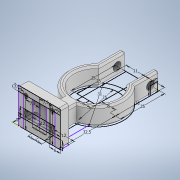
# Autodesk Inventor part: Endswitch Ender3 clamp
Saved by Autodesk Inventor 2020 (Build 240168000, 168)
## iProperties
Created: 2020-06-03
Part Number: Endswitch Ender3 clamp
Material: Generisch
Document SubType Name: Modeling
Designer: Daniel
Density: 1 g/cm^3
Appearance: Vorgabe
Author: Daniel
Autodesk Inventor part; units mm, degrees
ref_plane "YZ Plane" through (0, 0, 0) normal (1, 0, 0) x (0, 1, 0)
ref_plane "XZ Plane" through (0, 0, 0) normal (0, 1, 0) x (-1, 0, 0)
ref_plane "XY Plane" through (0, 0, 0) normal (0, 0, 1) x (1, 0, 0)
sketch "Skizze1" plane through (0, 0, 0) normal (0, 1, 0) x (-1, 0, 0)
  circle A0 centre (0, 0) radius 12.5
  line L0 (0, 0) -> (8, 0)
  line L1 (8, 0) -> (8, -25)
  line L2 (8, -25) -> (0, -25)
  line L3 (0, -25) -> (0, 0)
  line L4 (0, 0) -> (-8, 0)
  line L5 (-8, 0) -> (-8, -25)
  line L6 (-8, -25) -> (0, -25)
  line L7 (0, -25) -> (0, 0)
  line L8 (8, 0) -> (-8, 0)
  line L9 (-8, 0) -> (-8, 32.5)
  line L10 (-8, 32.5) -> (8, 32.5)
  line L11 (8, 32.5) -> (8, 0)
  line L12 (0, 32.5) -> (0, 27.5)
  line L13 (0, 27.5) -> (-12, 27.5)
  line L14 (-12, 27.5) -> (-12, 32.5)
  line L15 (-12, 32.5) -> (0, 32.5)
  line L16 (0, 32.5) -> (12, 32.5)
  line L17 (12, 32.5) -> (12, 27.5)
  line L18 (12, 27.5) -> (0, 27.5)
  line L19 (0, 27.5) -> (0, 32.5)
  circle A1 centre (0, 0) radius 15.5
  line L20 (0, 0) -> (11, 0)
  line L21 (11, 0) -> (11, -25)
  line L22 (11, -25) -> (0, -25)
  line L23 (0, -25) -> (0, 0)
  line L24 (0, 0) -> (-11, 0)
  line L25 (-11, 0) -> (-11, -25)
  line L26 (-11, -25) -> (0, -25)
  line L27 (0, -25) -> (0, 0)
  line L28 (0, 0) -> (4, 0)
  line L29 (4, 0) -> (4, 32.5)
  line L30 (4, 32.5) -> (0, 32.5)
  line L31 (0, 32.5) -> (0, 0)
  line L32 (0, 0) -> (-4, 0)
  line L33 (-4, 0) -> (-4, 32.5)
  line L34 (-4, 32.5) -> (0, 32.5)
  line L35 (0, 32.5) -> (0, 0)
  point P0 (8, -9.6047)
  point P1 (11, -10.9202)
  point P2 (4, 14.975)
  point P3 (4, 27.5)
  point P4 (-4, 27.5)
  point P5 (-4, 14.975)
  point P6 (-11, -10.9202)
  point P7 (-8, -9.6047)
  dimension "d0" = 25
  dimension "d1" = 8
  dimension "d2" = 25
  dimension "d3" = 8
  dimension "d4" = 25
  dimension "d5" = 32.5
  dimension "d6" = 5
  dimension "d7" = 12
  dimension "d8" = 12
  dimension "d9" = 5
  dimension "d10" = 31
  dimension "d11" = 11
  dimension "d12" = 25
  dimension "d13" = 11
  dimension "d14" = 25
  dimension "d15" = 4
  dimension "d16" = 4
  constraints: 72 end point, 19 parallel, 9 perpendicular, 7 horizontal, 3 point on line, 2 centre point, 2 coincident, 1 midpoint
  measures "d0" diameter of A0
  measures "d1" distance of L0.start L0.end
  measures "d2" distance of L0.end L1.end
  measures "d3" distance of L0.start L4.end
  measures "d4" distance of L5.end L4.end
  measures "d5" distance of L8.end L9.end
  measures "d6" distance of L12.start L12.end
  measures "d7" distance of L12.end L13.end
  measures "d8" distance of L17.end L18.end
  measures "d9" distance of L16.end L17.end
  measures "d10" diameter of A1
  measures "d11" distance of L21.end L22.end
  measures "d12" distance of L20.end L21.end
  measures "d13" distance of L26.end L25.end
  measures "d14" distance of L25.end L24.end
  measures "d15" distance of L30.end L29.end
  measures "d16" distance of L33.end L34.end
extrude "Extrusion1" add sketch "Skizze1" along normal blind 10 contours A0 L11 A1 L21 | A0 L29 A1 L11 | L21 A1 L1 A0 | A0 L31 A1 L29 | L21 L22 L1 A1 | A0 L33 A1 L31 | A1 L31 L18 L29 | A0 L9 A1 L33 | A1 L33 L13 L31 | L5 A1 L25 A0 | A0 L25 A1 L9 | L5 L26 L25 A1
extrude "Extrusion2" add sketch "Skizze1" along normal blind 20 separate body contours L18 L29 L10 L11 | L11 L16 L17 L18 | L18 L12 L10 L29 | L13 L33 L10 L12 | L13 L9 L10 L33 | L13 L14 L15 L9
sketch "Skizze2" plane through (-12, 0, 32.5) normal (0, 0, 1) x (1, 0, 0)
  line L0 (8, 0) -> (-3.5, 0) projected
  line L1 (-0.0236, 0) -> (23.9764, 0)
  line L2 (23.9764, 0) -> (23.9764, 5)
  line L3 (23.9764, 5) -> (-0.0236, 5)
  line L4 (-0.0236, 5) -> (-0.0236, 0)
  line L5 (0, 20) -> (24, 20) projected
  line L6 (-0.0236, 0) -> (2.9764, 0)
  line L7 (2.9764, 0) -> (2.9764, 17)
  line L8 (2.9764, 17) -> (-0.0236, 17)
  line L9 (-0.0236, 17) -> (-0.0236, 0)
  line L10 (23.9764, 0) -> (20.9764, 0)
  line L11 (20.9764, 0) -> (20.9764, 17)
  line L12 (20.9764, 17) -> (23.9764, 17)
  line L13 (23.9764, 17) -> (23.9764, 0)
  line L14 (24, 0) -> (24, 20) projected
  line L15 (24, 20) -> (18, 20)
  line L16 (18, 20) -> (18, 0)
  line L17 (18, 0) -> (24, 0)
  line L18 (24, 0) -> (24, 20)
  line L19 (24, 20) -> (-0.0236, 20)
  line L20 (-0.0236, 20) -> (-0.0236, 17)
  line L21 (-0.0236, 17) -> (24, 17)
  line L22 (24, 17) -> (24, 20)
  line L23 (11.9882, 17) -> (15.9882, 17)
  line L24 (15.9882, 17) -> (15.9882, 5)
  line L25 (15.9882, 5) -> (11.9882, 5)
  line L26 (11.9882, 5) -> (11.9882, 17)
  line L27 (11.9882, 17) -> (7.9882, 17)
  line L28 (7.9882, 17) -> (7.9882, 5)
  line L29 (7.9882, 5) -> (11.9882, 5)
  line L30 (11.9882, 5) -> (11.9882, 17)
  line L31 (20.9764, 5) -> (2.9764, 5)
  line L32 (2.9764, 5) -> (2.9764, 10)
  line L33 (2.9764, 10) -> (20.9764, 10)
  line L34 (20.9764, 10) -> (20.9764, 5)
  line L35 (11.9882, 17) -> (4.4882, 17)
  line L36 (11.9882, 17) -> (19.4882, 17)
  point P0 (12, 0)
  point P1 (1, 0)
  point P2 (15.9882, 10)
  point P3 (7.9882, 10)
  dimension "d21" = 24
  dimension "d22" = 5
  dimension "d24" = 3
  dimension "d25" = 17
  dimension "d26" = 3
  dimension "d27" = 17
  dimension "d35" = 6
  dimension "d36" = 3
  dimension "d37" = 4
  dimension "d38" = 4
  dimension "d41" = 5
  dimension "d55" = 7.5
  dimension "d56" = 7.5
  constraints: 68 end point, 16 parallel, 9 point on line, 8 horizontal, 8 perpendicular, 1 midpoint
  measures "d21" distance of L3.end L2.end
  measures "d22" distance of L2.end L1.end
  measures "d24" distance of L8.end L7.end
  measures "d25" distance of L7.end L6.end
  measures "d26" distance of L11.end L12.end
  measures "d27" distance of L10.end L11.end
  measures "d35" distance of L17.end L16.end
  measures "d36" distance of L8.end L19.end
  measures "d37" distance of L24.end L25.end
  measures "d38" distance of L29.end L28.end
  measures "d41" distance of L31.end L32.end
  measures "d55" distance of L23.start L35.end
  measures "d56" distance of L23.start L36.end
extrude "Extrusion3" cut sketch "Skizze2" against normal blind 3 contours L7 L33 L28 L3 | L16 L33 L11 L3 | L3 L24 L33 L16 | L28 L33 L26 L3 | L3 L26 L33 L24 | L28 L21 L26 L33 | L33 L26 L21 L24 bodies 2
fillet "Rundung1" radius 2 8 edges at (-9.0236, 7.5, 29.5) (-0.0236, 5, 29.5) (-4.0118, 13.5, 29.5) (-0.0118, 17, 29.5) (-6.5177, 10, 29.5) (6.4823, 10, 29.5) (3.9882, 13.5, 29.5) (8.9764, 7.5, 29.5)
chamfer "Fase1" distance 1 angle 45 30 edges at (0, 10, 12.5) (-8, 10, -17.3023) (8, 10, -17.3023) (11, 10, -17.9601) (14.9629, 10, 4.0448) (4, 10, 21.2375) (-4, 10, 21.2375) (-14.9629, 10, 4.0448) (-11, 10, -17.9601) (4, 0, 21.2375) (14.9629, 0, 4.0448) (11, 0, -17.9601) (-11, 0, -17.9601) (-14.9629, 0, 4.0448) (-4, 0, 21.2375) (0, 0, 12.5) (-8, 0, -17.3023) (8, 0, -17.3023) (-8, 5, -25) (11, 5, -25) (-11, 5, -25) (9.5, 10, -25) (-9.5, 10, -25) (9.5, 0, -25) (-9.5, 0, -25) (8, 5, -25) (12, 20, 30) (-12, 20, 30) (12, 0, 30) (-12, 0, 30)
sketch "Skizze3" plane through (11, 1, -10.9202) normal (1, 0, 0) x (0, 0, -1)
  line L0 (13.0798, -1) -> (14.0798, 0) projected
  line L1 (13.0798, -1) -> (9.0798, -1)
  line L2 (9.0798, -1) -> (9.0798, 4)
  line L3 (9.0798, 4) -> (13.0798, 4)
  line L4 (13.0798, 4) -> (13.0798, -1)
  point P0 (-10.9202, -1)
  dimension "d46" = 4
  dimension "d47" = 5
  constraints: 8 end point, 2 parallel, 1 horizontal, 1 perpendicular
  measures "d46" distance of L2.end L3.end
  measures "d47" distance of L1.end L2.end
hole "Bohrung2" at (11, 5, -20) direction (-1, 0, 0) diameter 4.5 end through all bodies 1 clearance for "Flachkopfsenkschraube ISO 2009/7046" size "M4" standard "ISO"
hole "Bohrung3" at (-7.5118, 17, 32.5) at (7.4882, 17, 32.5) direction (0, 0, -1) diameter 2.459 end through all bodies 2 thread size "M3x0.5" class "6H" standard "ISO Metric profile"
